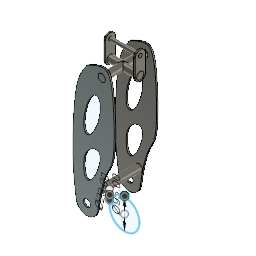
Assembly (Autodesk Fusion 360 archive; units mm, degrees)
design "Upper Leg 2"
Autodesk Fusion 360 part; units mm, degrees
sketch "Sketch1" plane through (0, 0, 0) normal (0, 1, 0) x (1, 0, 0)
  circle A0 centre (0, 0) radius 11.5
  line L0 (0, 0) -> (0, -380) construction
  spline S0 degree 5 poles (-34.999996, 0.018371) (-36.765337, -11.793617) (-39.872399, -35.13832) (-43.262167, -69.317601) (-45.439734, -113.053889) (-45.27808, -163.764753) (-43.38331, -209.425485) (-40.662731, -249.125572) (-37.474948, -282.5252) (-33.177392, -310.465503) (-25.886685, -335.507594) (-17.30111, -354.014091) (-9.259092, -367.256165) (-3.202461, -375.799306) (0, -380) knots 0 0 0 0 0 0 0.1 0.2 0.3 0.4 0.5 0.6 0.7 0.8 0.9 1 1 1 1 1 1
  spline S1 degree 5 poles (34.515327, 5.804498) (35.963743, -4.372947) (38.918644, -23.706579) (43.525767, -49.639335) (50.015767, -78.070342) (58.632078, -103.722208) (67.407218, -121.676463) (75.78372, -135.624073) (82.448877, -154.607429) (86.321684, -186.28222) (87.534612, -229.207065) (86.474743, -278.560732) (83.560554, -326.813369) (78.68464, -366.51809) (70.877846, -391.915922) (57.645781, -401.754153) (40.264756, -398.566887) (22.222842, -391.087647) (7.805787, -384.039611) (0, -380) knots 0 0 0 0 0 0 0.06666667 0.13333333 0.2 0.26666667 0.33333333 0.4 0.46666667 0.53333333 0.6 0.66666667 0.73333333 0.8 0.86666667 0.93333333 1 1 1 1 1 1
  line L1 (-40.249082, -261.962022) -> (-31.187007, -321.771715)
  line L2 (-27.331562, 51.328246) -> (-42.668428, -51.291504)
  line L3 (66.819635, -116.599811) -> (84.627241, -158.85584)
  line L4 (84.763476, -342.482965) -> (65.236524, -407.517035)
  line L5 (-24.170199, -348.295747) -> (24.170199, -411.704253)
  line L6 (73.364414, -417.967179) -> (-73.364414, -342.032821)
  arc A1 (34.758913, 4.10098) -> (-34.999996, 0.018358) centre (0, 0) ccw
  spline S2 degree 5 poles (30.559346, -310.688008) (29.218041, -310.842547) (26.407033, -310.584734) (21.871267, -308.49137) (15.460511, -302.375191) (7.547525, -289.881367) (0.418087, -273.62641) (-5.307828, -255.024034) (-9.114425, -235.748931) (-10.635493, -217.687449) (-9.675031, -202.729791) (-6.22928, -192.54826) (-0.514164, -188.374513) (7.003778, -190.767494) (15.569514, -199.364673) (24.263427, -213.106469) (32.121219, -230.450327) (38.258773, -249.577012) (41.984579, -268.582655) (42.950446, -285.689465) (41.187656, -299.383866) (37.835055, -306.648833) (34.454865, -309.657497) (31.900652, -310.533468) (30.559346, -310.688008) knots 0 0 0 0 0 0 0.05 0.1 0.15 0.2 0.25 0.3 0.35 0.4 0.45 0.5 0.55 0.6 0.65 0.7 0.75 0.8 0.85 0.9 0.95 1 1 1 1 1 1
  spline S3 degree 5 poles (12.77765, -155.473996) (11.061501, -154.198275) (7.722893, -151.4254) (3.092974, -146.686647) (-2.060882, -139.418143) (-6.592091, -128.902644) (-9.288799, -117.003879) (-10.351176, -103.9516) (-9.964712, -90.392036) (-8.106168, -77.772161) (-4.580124, -68.140656) (0.762081, -63.484888) (7.8759, -65.257609) (16.29499, -73.686842) (25.098061, -87.602596) (33.14979, -104.991619) (39.275614, -123.365054) (42.455308, -140.176433) (42.027621, -153.237866) (37.861606, -161.083892) (30.646713, -163.518201) (23.492918, -161.825575) (18.019788, -159.079725) (14.4938, -156.749717) (12.77765, -155.473996) knots 0 0 0 0 0 0 0.05 0.1 0.15 0.2 0.25 0.3 0.35 0.4 0.45 0.5 0.55 0.6 0.65 0.7 0.75 0.8 0.85 0.9 0.95 1 1 1 1 1 1
  point P0 (-35.718045, -291.866868)
  point P1 (75.723438, -137.727826)
  point P2 (75, -375)
  point P3 (-5.21469, -253.298202)
  point P4 (0, -190)
  point P5 (40, -260)
  point P6 (-10, -98.170733)
  point P7 (5.172689, -65.386568)
  point P8 (40, -155.473996)
  dimension "d1" = 23
  dimension "d2" = 70
  dimension "d3" = 380
  constraint coincident A0.centre L0.start
  constraint vertical L0
  constraint midpoint P2 L4
  constraint midpoint L0.end L5
  constraint midpoint L0.end L6
  constraint midpoint L0 P4
  measures "d1" diameter of A0
  measures "d2" diameter of A1
  measures "d3" distance of A0.centre L0.end
extrude "Extrude1" add sketch "Sketch1" along normal blind 5 contours S0 S1 L2 A1 | L2 A1 picked at (44.211523, -353.089122) picked at (-34.264893, 5.702053) makes body 1
ref_plane "WorkPlane1" through (0, 70, 0) normal (0, 1, 0) x (0, 0, 1)
mirror "Mirror1" about plane through (0, 70, 0) normal (0, 1, 0) of bodies 1 makes body 2
copy_body "CutPasteBodies1" bodies 1 removing the originals makes body 3 in component "Link 1"
copy_body "CutPasteBodies2" bodies 2 removing the originals makes body 4 in component "Link 1"
sketch "Sketch2" plane through (0, 5, 0) normal (0, 1, 0) x (-1, 0, 0)
  spline S0 degree 5 poles (-30.559346, 310.688008) (-29.218041, 310.842547) (-26.407033, 310.584734) (-21.871267, 308.49137) (-15.460511, 302.375191) (-7.547525, 289.881367) (-0.418087, 273.62641) (5.307828, 255.024034) (9.114425, 235.748931) (10.635493, 217.687449) (9.675031, 202.729791) (6.22928, 192.54826) (0.514164, 188.374513) (-7.003778, 190.767494) (-15.569514, 199.364673) (-24.263427, 213.106469) (-32.121219, 230.450327) (-38.258773, 249.577012) (-41.984579, 268.582655) (-42.950446, 285.689465) (-41.187656, 299.383866) (-37.835055, 306.648833) (-34.454865, 309.657497) (-31.900652, 310.533468) (-30.559346, 310.688008) knots 0 0 0 0 0 0 0.05 0.1 0.15 0.2 0.25 0.3 0.35 0.4 0.45 0.5 0.55 0.6 0.65 0.7 0.75 0.8 0.85 0.9 0.95 1 1 1 1 1 1
  spline S1 degree 5 poles (-12.77765, 155.473996) (-11.061501, 154.198275) (-7.722893, 151.4254) (-3.092974, 146.686647) (2.060882, 139.418143) (6.592091, 128.902644) (9.288799, 117.003879) (10.351176, 103.9516) (9.964712, 90.392036) (8.106168, 77.772161) (4.580124, 68.140656) (-0.762081, 63.484888) (-7.8759, 65.257609) (-16.29499, 73.686842) (-25.098061, 87.602596) (-33.14979, 104.991619) (-39.275614, 123.365054) (-42.455308, 140.176433) (-42.027621, 153.237866) (-37.861606, 161.083892) (-30.646713, 163.518201) (-23.492918, 161.825575) (-18.019788, 159.079725) (-14.4938, 156.749717) (-12.77765, 155.473996) knots 0 0 0 0 0 0 0.05 0.1 0.15 0.2 0.25 0.3 0.35 0.4 0.45 0.5 0.55 0.6 0.65 0.7 0.75 0.8 0.85 0.9 0.95 1 1 1 1 1 1
  circle A0 centre (0, 0) radius 11.5
  spline S2 degree 5 poles (34.999996, -0.018371) (36.765337, 11.793617) (39.872399, 35.13832) (43.262167, 69.317601) (45.439734, 113.053889) (45.27808, 163.764753) (43.38331, 209.425485) (40.662731, 249.125572) (37.474948, 282.5252) (33.177392, 310.465503) (25.886685, 335.507594) (17.30111, 354.014091) (9.259092, 367.256165) (3.202461, 375.799306) (0, 380) knots 0 0 0 0 0 0 0.1 0.2 0.3 0.4 0.5 0.6 0.7 0.8 0.9 1 1 1 1 1 1
  spline S3 degree 5 poles (0, 380) (-7.805787, 384.039611) (-22.222842, 391.087647) (-40.264756, 398.566887) (-57.645781, 401.754153) (-70.877846, 391.915922) (-78.68464, 366.51809) (-83.560554, 326.813369) (-86.474743, 278.560732) (-87.534612, 229.207065) (-86.321684, 186.28222) (-82.448877, 154.607429) (-75.78372, 135.624073) (-67.407218, 121.676463) (-58.632078, 103.722208) (-50.073651, 78.242669) (-43.634794, 50.11627) (-39.073493, 24.575916) (-36.162448, 5.668302) (-34.758913, -4.10098) knots -1 -1 -1 -1 -1 -1 -0.93333333 -0.86666667 -0.8 -0.73333333 -0.66666667 -0.6 -0.53333333 -0.46666667 -0.4 -0.33333333 -0.26666667 -0.2 -0.13333333 -0.06666667 -0.0022393 -0.0022393 -0.0022393 -0.0022393 -0.0022393 -0.0022393
  spline S4 degree 5 poles (-34.758913, -4.10098) (-34.71013, -4.440531) (-34.66138, -4.780659) (-34.612663, -5.121362) (-34.563979, -5.462642) (-34.515327, -5.804498) knots -0.0022393 -0.0022393 -0.0022393 -0.0022393 -0.0022393 -0.0022393 0 0 0 0 0 0
  arc A1 (-34.515328, -5.804498) -> (34.999996, -0.018371) centre (0, 0) ccw
  line L0 (-37.495253, 64.762358) -> (-18.477431, 23.978508)
  line L1 (-18.477431, 23.978508) -> (-23.00897, 21.865417)
  line L2 (-23.00897, 21.865417) -> (-42.026792, 62.649267)
  line L3 (-42.026792, 62.649267) -> (-37.495253, 64.762358)
  circle A2 centre (-30, 45) radius 11.5
  dimension "d9" = 45
  dimension "d10" = 5
  dimension "d83" = 23
  measures "d83" diameter of A2
extrude "Extrude1'" add sketch "Sketch2" along normal blind 135 contours L0 A2 | L0 L2 A2 | L2 A2 picked at (-25.201363, 48.418586) picked at (-31.643456, 48.269471) picked at (-34.932087, 40.620912) bodies 4 3 in component "Link 1"
sketch "Sketch3" plane through (0, 0, 0) normal (0, -1, 0) x (1, 0, 0)
  spline S0 degree 5 poles (30.559346, 310.688008) (29.218041, 310.842547) (26.407033, 310.584734) (21.871267, 308.49137) (15.460511, 302.375191) (7.547525, 289.881367) (0.418087, 273.62641) (-5.307828, 255.024034) (-9.114425, 235.748931) (-10.635493, 217.687449) (-9.675031, 202.729791) (-6.22928, 192.54826) (-0.514164, 188.374513) (7.003778, 190.767494) (15.569514, 199.364673) (24.263427, 213.106469) (32.121219, 230.450327) (38.258773, 249.577012) (41.984579, 268.582655) (42.950446, 285.689465) (41.187656, 299.383866) (37.835055, 306.648833) (34.454865, 309.657497) (31.900652, 310.533468) (30.559346, 310.688008) knots 0 0 0 0 0 0 0.05 0.1 0.15 0.2 0.25 0.3 0.35 0.4 0.45 0.5 0.55 0.6 0.65 0.7 0.75 0.8 0.85 0.9 0.95 1 1 1 1 1 1
  spline S1 degree 5 poles (12.77765, 155.473996) (11.061501, 154.198275) (7.722893, 151.4254) (3.092974, 146.686647) (-2.060882, 139.418143) (-6.592091, 128.902644) (-9.288799, 117.003879) (-10.351176, 103.9516) (-9.964712, 90.392036) (-8.106168, 77.772161) (-4.580124, 68.140656) (0.762081, 63.484888) (7.8759, 65.257609) (16.29499, 73.686842) (25.098061, 87.602596) (33.14979, 104.991619) (39.275614, 123.365054) (42.455308, 140.176433) (42.027621, 153.237866) (37.861606, 161.083892) (30.646713, 163.518201) (23.492918, 161.825575) (18.019788, 159.079725) (14.4938, 156.749717) (12.77765, 155.473996) knots 0 0 0 0 0 0 0.05 0.1 0.15 0.2 0.25 0.3 0.35 0.4 0.45 0.5 0.55 0.6 0.65 0.7 0.75 0.8 0.85 0.9 0.95 1 1 1 1 1 1
  circle A0 centre (0, 0) radius 11.5
  spline S2 degree 5 poles (-34.999996, -0.018371) (-36.765337, 11.793617) (-39.872399, 35.13832) (-43.262167, 69.317601) (-45.439734, 113.053889) (-45.27808, 163.764753) (-43.38331, 209.425485) (-40.662731, 249.125572) (-37.474948, 282.5252) (-33.177392, 310.465503) (-25.886685, 335.507594) (-17.30111, 354.014091) (-9.259092, 367.256165) (-3.202461, 375.799306) (0, 380) knots 0 0 0 0 0 0 0.1 0.2 0.3 0.4 0.5 0.6 0.7 0.8 0.9 1 1 1 1 1 1
  arc A1 (-34.999996, -0.018371) -> (34.515328, -5.804498) centre (0, 0) ccw
  spline S3 degree 5 poles (34.515327, -5.804498) (34.563979, -5.462642) (34.612663, -5.121362) (34.66138, -4.780659) (34.71013, -4.440531) (34.758913, -4.10098) knots 0 0 0 0 0 0 0.0022393 0.0022393 0.0022393 0.0022393 0.0022393 0.0022393
  spline S4 degree 5 poles (34.758913, -4.10098) (36.162448, 5.668302) (39.073493, 24.575916) (43.634794, 50.11627) (50.073651, 78.242669) (58.632078, 103.722208) (67.407218, 121.676463) (75.78372, 135.624073) (82.448877, 154.607429) (86.321684, 186.28222) (87.534612, 229.207065) (86.474743, 278.560732) (83.560554, 326.813369) (78.68464, 366.51809) (70.877846, 391.915922) (57.645781, 401.754153) (40.264756, 398.566887) (22.222842, 391.087647) (7.805787, 384.039611) (0, 380) knots 0.0022393 0.0022393 0.0022393 0.0022393 0.0022393 0.0022393 0.06666667 0.13333333 0.2 0.26666667 0.33333333 0.4 0.46666667 0.53333333 0.6 0.66666667 0.73333333 0.8 0.86666667 0.93333333 1 1 1 1 1 1
  circle A2 centre (47.488742, 368.730489) radius 11.5
  dimension "d13" = 23
  measures "d13" diameter of A2
extrude "Extrude2" cut sketch "Sketch3" against normal blind 190 contours A2 picked at (50.698805, 365.999766) bodies 4 in component "Link 1"
extrude "Extrude1''" add sketch "Sketch3" along normal blind -140 and the other way blind 5 separate body contours A2 picked at (50.698805, 365.999766) makes body 5 in component "Hooks Joint"
copy_body "CopyPasteBodies1" bodies 5 makes body 6 in component "Hooks Joint"
move_body "Move1" bodies 6 to x (1, 0, 0) y (0, 0, 1) z (0, -1, 0) at (0, 397.230489, 337.230489) in component "Hooks Joint"
ref_plane "WorkPlane1" through (47.488742, 72.5, 368.730489) normal (0, -1, 0) x (1, 0, 0) in component "Hooks Joint"
sketch "Sketch4" plane through (47.488742, 72.5, 368.730489) normal (0, -1, 0) x (1, 0, 0)
  circle A0 through (0, -11.5, 0) (0, 5.75, 9.959292) (0, 5.75, -9.959292)
  dimension "d20" = 23
extrude "Extrude2'" add sketch "Sketch4" along normal blind 55 and the other way blind 45 contours A0 in plane through (47.488742, 72.5, 368.730489) normal (1, 0, 0) picked at (47.488742, 73.219113, 371.540521) bodies 5 in component "Hooks Joint"
sketch "Sketch5" plane through (2.488742, 0, 0) normal (-1, 0, 0) x (0, -1, 0)
  circle A0 centre (-72.5, 368.730489) radius 11.5
  circle A1 centre (-72.5, 368.730489) radius 12.5
  dimension "d25" = 1
extrude "Extrude1'''" add sketch "Sketch5" against normal blind 5 separate body contours A1 picked at (-70.974989, 380.770319) makes body 7 in component "second ling"
sketch "Sketch6" plane through (2.488742, 0, 0) normal (-1, 0, 0) x (0, -1, 0)
  circle A0 centre (-72.5, 368.730489) radius 11.5
  circle A1 centre (-72.5, 368.730489) radius 12.5
  line L0 (-72.5, 368.730489) -> (-72.5, 430) construction
  line L1 (-72.5, 423.730489) -> (-37.000001, 423.730489)
  line L2 (-56.136364, 368.730489) -> (-56.136364, 423.730489)
  arc A2 (-56.136364, 423.730489) -> (-88.863636, 423.730489) centre (-72.5, 423.730489) ccw
  line L3 (-88.863636, 423.730489) -> (-88.863636, 368.730489)
  arc A3 (-88.863636, 368.730489) -> (-56.136364, 368.730489) centre (-72.5, 368.730489) ccw
  line L4 (-72.5, 368.730489) -> (-72.5, 423.730489) construction
  circle A4 centre (-72.5, 368.730489) radius 12.5
  circle A5 centre (-72.5, 423.730489) radius 6
  dimension "d32" = 12
  dimension "d33" = 55
  constraint vertical L0
  constraint perpendicular L0 L1
  constraint tangent L2 A2
  constraint tangent A2 L3
  constraint parallel L2 L3
  constraint tangent L3 A3
  constraint tangent L2 A3
  constraint perpendicular L1 L4
  constraint concentric A2 A5
  measures "d32" diameter of A5
extrude "Extrude3" add sketch "Sketch6" against normal blind 5 contours L2 A2 L3 A3 picked at (-63.715142, 407.441932) bodies 7 in component "second ling"
copy_body "CopyPasteBodies1'" bodies 7 makes body 8
move_body "Move1'" bodies 8 to x (1, 0, 0) y (0, 1, 0) z (0, 0, 1) at (95, 0, 0)
extrude "Extrude4" add sketch "Sketch6" against normal blind 100 contours A5 picked at (-72.945042, 428.80767) bodies 7 in component "second ling"
ref_plane "WorkPlane2" through (52.488742, 72.5, 396.230489) normal (-1, 0, 0) x (0, -1, 0)
ref_plane "WorkPlane3" through (46.760421, 72.5, 429.730489) normal (0, 0, 1) x (0, 1, 0)
sketch "Sketch9" plane through (46.760421, 30, 429.730489) normal (0, 0, 1) x (1, 0, 0)
  circle A0 centre (0.73, 0) radius 6
  dimension "d37" = 12
  measures "d37" diameter of A0
sketch "Sketch1 (2)" plane through (0, 5, 0) normal (0, -1, 0) x (1, 0, 0) in component "Gear\\"
  circle A0 centre (47.488742, 368.730489) radius 11.5
  spline S0 degree 5 poles (30.559346, 310.688008) (29.218041, 310.842547) (26.407033, 310.584734) (21.871267, 308.49137) (15.460511, 302.375191) (7.547525, 289.881367) (0.418087, 273.62641) (-5.307828, 255.024034) (-9.114425, 235.748931) (-10.635493, 217.687449) (-9.675031, 202.729791) (-6.22928, 192.54826) (-0.514164, 188.374513) (7.003778, 190.767494) (15.569514, 199.364673) (24.263427, 213.106469) (32.121219, 230.450327) (38.258773, 249.577012) (41.984579, 268.582655) (42.950446, 285.689465) (41.187656, 299.383866) (37.835055, 306.648833) (34.454865, 309.657497) (31.900652, 310.533468) (30.559346, 310.688008) knots 0 0 0 0 0 0 0.05 0.1 0.15 0.2 0.25 0.3 0.35 0.4 0.45 0.5 0.55 0.6 0.65 0.7 0.75 0.8 0.85 0.9 0.95 1 1 1 1 1 1
  spline S1 degree 5 poles (12.77765, 155.473996) (11.061501, 154.198275) (7.722893, 151.4254) (3.092974, 146.686647) (-2.060882, 139.418143) (-6.592091, 128.902644) (-9.288799, 117.003879) (-10.351176, 103.9516) (-9.964712, 90.392036) (-8.106168, 77.772161) (-4.580124, 68.140656) (0.762081, 63.484888) (7.8759, 65.257609) (16.29499, 73.686842) (25.098061, 87.602596) (33.14979, 104.991619) (39.275614, 123.365054) (42.455308, 140.176433) (42.027621, 153.237866) (37.861606, 161.083892) (30.646713, 163.518201) (23.492918, 161.825575) (18.019788, 159.079725) (14.4938, 156.749717) (12.77765, 155.473996) knots 0 0 0 0 0 0 0.05 0.1 0.15 0.2 0.25 0.3 0.35 0.4 0.45 0.5 0.55 0.6 0.65 0.7 0.75 0.8 0.85 0.9 0.95 1 1 1 1 1 1
  circle A1 centre (0, 0) radius 11.5
  spline S2 degree 5 poles (-34.999996, -0.018371) (-36.765337, 11.793617) (-39.872399, 35.13832) (-43.262167, 69.317601) (-45.439734, 113.053889) (-45.27808, 163.764753) (-43.38331, 209.425485) (-40.662731, 249.125572) (-37.474948, 282.5252) (-33.177392, 310.465503) (-25.886685, 335.507594) (-17.30111, 354.014091) (-9.259092, 367.256165) (-3.202461, 375.799306) (0, 380) knots 0 0 0 0 0 0 0.1 0.2 0.3 0.4 0.5 0.6 0.7 0.8 0.9 1 1 1 1 1 1
  arc A2 (-34.999996, -0.018371) -> (34.515328, -5.804498) centre (0, 0) ccw
  spline S3 degree 5 poles (34.515327, -5.804498) (34.563979, -5.462642) (34.612663, -5.121362) (34.66138, -4.780659) (34.71013, -4.440531) (34.758913, -4.10098) knots 0 0 0 0 0 0 0.0022393 0.0022393 0.0022393 0.0022393 0.0022393 0.0022393
  spline S4 degree 5 poles (34.758913, -4.10098) (36.162448, 5.668302) (39.073493, 24.575916) (43.634794, 50.11627) (50.073651, 78.242669) (58.632078, 103.722208) (67.407218, 121.676463) (75.78372, 135.624073) (82.448877, 154.607429) (86.321684, 186.28222) (87.534612, 229.207065) (86.474743, 278.560732) (83.560554, 326.813369) (78.68464, 366.51809) (70.877846, 391.915922) (57.645781, 401.754153) (40.264756, 398.566887) (22.222842, 391.087647) (7.805787, 384.039611) (0, 380) knots 0.0022393 0.0022393 0.0022393 0.0022393 0.0022393 0.0022393 0.06666667 0.13333333 0.2 0.26666667 0.33333333 0.4 0.46666667 0.53333333 0.6 0.66666667 0.73333333 0.8 0.86666667 0.93333333 1 1 1 1 1 1
  circle A3 centre (72.000001, 44.999966) radius 11.5
  line L0 (72.000001, 44.999966) -> (72.000001, 75.000001) construction
  spline S5 degree 5 poles (70.676203, 56.423519) (70.740357, 56.505992) (70.861965, 56.667998) (71.02428, 56.90218) (71.19983, 57.196473) (71.348048, 57.532916) (71.422976, 57.836587) (71.427557, 58.107869) (71.373553, 58.350404) (71.289923, 58.574495) (71.218824, 58.795588) (71.206768, 58.982847) (71.238957, 59.13501) (71.280896, 59.242445) (71.306987, 59.297662) knots 0 0 0 0 0 0 0.1 0.2 0.3 0.4 0.5 0.6 0.7 0.8 0.9 1 1 1 1 1 1
  line L1 (71.14471, 58.954229) -> (71.469264, 59.641095)
  spline S6 degree 5 poles (71.306987, 59.297662) (71.324621, 59.340885) (71.364787, 59.41941) (71.439713, 59.513463) (71.563314, 59.597873) (71.732716, 59.65742) (71.8588, 59.681782) (71.937248, 59.690725) (71.980579, 59.692713) (72.000001, 59.692713) knots 0 0 0 0 0 0 0.2 0.4 0.6 0.8 1 1 1 1 1 1
  line L2 (71.949992, 59.692713) -> (72.05001, 59.692713)
  line L3 (71.263265, 59.190493) -> (71.35071, 59.404831)
  spline S7 degree 5 poles (73.323799, 56.423519) (73.259645, 56.505992) (73.138037, 56.667998) (72.975722, 56.90218) (72.800172, 57.196473) (72.651954, 57.532916) (72.577026, 57.836587) (72.572445, 58.107869) (72.626449, 58.350404) (72.710079, 58.574495) (72.781178, 58.795588) (72.793234, 58.982847) (72.761045, 59.13501) (72.719106, 59.242445) (72.693015, 59.297662) knots 0 0 0 0 0 0 0.1 0.2 0.3 0.4 0.5 0.6 0.7 0.8 0.9 1 1 1 1 1 1
  line L4 (70.395037, 56.06206) -> (70.95737, 56.784977)
  line L5 (73.604965, 56.06206) -> (73.042632, 56.784977)
  line L6 (72.855292, 58.954229) -> (72.530738, 59.641095)
  spline S8 degree 5 poles (72.693015, 59.297662) (72.675381, 59.340885) (72.635216, 59.41941) (72.560289, 59.513463) (72.436688, 59.597873) (72.267286, 59.65742) (72.141202, 59.681782) (72.062754, 59.690725) (72.019423, 59.692713) (72.000001, 59.692713) knots 0 0 0 0 0 0 0.2 0.4 0.6 0.8 1 1 1 1 1 1
  line L7 (72.736737, 59.190493) -> (72.649293, 59.404831)
  line L8 (72.05001, 59.692713) -> (71.949992, 59.692713)
  circle A4 centre (119.753744, 29.801356) radius 47.5
  spline S9 degree 5 poles (121.122284, 77.285686) (121.05813, 77.36816) (120.936522, 77.530165) (120.774207, 77.764347) (120.598657, 78.05864) (120.450439, 78.395083) (120.375511, 78.698754) (120.37093, 78.970036) (120.424934, 79.212571) (120.508564, 79.436662) (120.579663, 79.657755) (120.591719, 79.845015) (120.55953, 79.997177) (120.517591, 80.104613) (120.4915, 80.159829) knots 0 0 0 0 0 0 0.1 0.2 0.3 0.4 0.5 0.6 0.7 0.8 0.9 1 1 1 1 1 1
  line L9 (121.40345, 76.924227) -> (120.841117, 77.647144)
  line L10 (120.653777, 79.816396) -> (120.329223, 80.503263)
  spline S10 degree 5 poles (120.4915, 80.159829) (120.473866, 80.203052) (120.433701, 80.281578) (120.358774, 80.37563) (120.235173, 80.46004) (120.065771, 80.519587) (119.939687, 80.543949) (119.861239, 80.552892) (119.817908, 80.55488) (119.798486, 80.55488) knots 0 0 0 0 0 0 0.2 0.4 0.6 0.8 1 1 1 1 1 1
  line L11 (120.535222, 80.052661) -> (120.447778, 80.266998)
  line L12 (119.848495, 80.55488) -> (119.748477, 80.55488)
  spline S11 degree 5 poles (118.474688, 77.285686) (118.538842, 77.36816) (118.66045, 77.530165) (118.822765, 77.764347) (118.998315, 78.05864) (119.146533, 78.395083) (119.221461, 78.698754) (119.226042, 78.970036) (119.172038, 79.212571) (119.088408, 79.436662) (119.017309, 79.657755) (119.005253, 79.845015) (119.037442, 79.997177) (119.079381, 80.104613) (119.105472, 80.159829) knots 0 0 0 0 0 0 0.1 0.2 0.3 0.4 0.5 0.6 0.7 0.8 0.9 1 1 1 1 1 1
  line L13 (118.193522, 76.924227) -> (118.755855, 77.647144)
  line L14 (118.943195, 79.816396) -> (119.26775, 80.503263)
  spline S12 degree 5 poles (119.105472, 80.159829) (119.123106, 80.203052) (119.163272, 80.281578) (119.238198, 80.37563) (119.361799, 80.46004) (119.531201, 80.519587) (119.657285, 80.543949) (119.735733, 80.552892) (119.779064, 80.55488) (119.798486, 80.55488) knots 0 0 0 0 0 0 0.2 0.4 0.6 0.8 1 1 1 1 1 1
  line L15 (119.06175, 80.052661) -> (119.149195, 80.266998)
  line L16 (119.748477, 80.55488) -> (119.848495, 80.55488)
  point P0 (71.399905, 58.200013)
  point P1 (72.600097, 58.200013)
  point P2 (119.19839, 79.06218)
  point P3 (120.398582, 79.06218)
  dimension "d84" = 23
  dimension "d99" = 95
  constraint vertical L0
  measures "d84" diameter of A3
  measures "d99" diameter of A4
extrude "Extrude1''''" [suppressed] in component "Gear\\"
pattern_circular "C-Pattern1" [suppressed] in component "Gear\\"
copy_body "CopyPasteBodies1''" [suppressed] in component "Gear 2"
move_body "Move1''" [suppressed] in component "Gear 2"
extrude "Extrude1'''''" [suppressed] in component "Gear 2"
component "Link 1" placed x (1, 0, 0) y (0, 1, 0) z (0, 0, 1) at (0, 5, 0)
component "Hooks Joint" placed x (1, 0, 0) y (0, 1, 0) z (0, 0, 1) at (0, 0, 0)
component "Gear\\" placed x (1, 0, 0) y (0, 1, 0) z (0, 0, 1) at (-42.000001, 122, 0.000034)
component "second ling" placed x (1, 0, 0) y (0, 1, 0) z (0, 0, 1) at (0, 0, 0) in component "Hooks Joint"
hidden bodies 6
